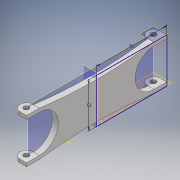
# Autodesk Inventor part: base
Saved by Autodesk Inventor 2017 (Build 210142000, 142)
## iProperties
Created: 2017-06-21
Part Number: base
Material: Generic
Document SubType Name: Modeling
Designer: erwin
Density: 1 g/cm^3
Appearance: Default
Author: erwin
Autodesk Inventor part; units mm, degrees
ref_plane "YZ Plane" through (0, 0, 0) normal (1, 0, 0) x (0, 1, 0)
ref_plane "XY Plane" through (0, 0, 0) normal (0, 0, 1) x (1, 0, 0)
ref_plane "Work Plane1" through (99, 43.8269, 0) normal (0, 0, 1) x (1, 0, 0)
sketch "Sketch1" plane through (99, 43.8269, 0) normal (0, 0, 1) x (1, 0, 0)
  circle A0 centre (13, 63.5) radius 3 projected
  arc A1 (20, 64) -> (13, 71) centre (13, 64) ccw projected
  line L0 (6, 71) -> (13, 71) projected
  arc A2 (2, 73) -> (6, 71) centre (6, 76) ccw projected
  line L1 (2, 71) -> (2, 73) projected
  line L2 (0, 71) -> (2, 71) projected
  line L3 (0, -43.8269) -> (0, 71) projected
  line L4 (-99, 0) -> (2, 0) projected
  line L5 (2, 56) -> (2, 0) projected
  line L6 (2, 56) -> (13, 56) projected
  arc A3 (13, 56) -> (20, 63) centre (13, 63) ccw projected
  line L7 (20, 64) -> (20, 63) projected
  circle A4 centre (13, 63.5) radius 3
  line L8 (6, 56) -> (21, 56)
  line L9 (21, 56) -> (21, 71)
  line L10 (21, 71) -> (6, 71)
  line L11 (6, 56) -> (20, 56)
  line L12 (20, 71) -> (6, 71)
  line L13 (6, 71) -> (6, 56)
  point P0 (-99, -43.8269)
  constraints: 12 end point, 2 horizontal, 2 parallel, 2 point on circle, 1 centre point, 1 coincident, 1 concentric, 1 perpendicular, 1 point on line
extrude "Extrusion1" add sketch "Sketch1" along normal blind 4 contours L7 A3 L6 L13 L0 A1 | A1 L10 L9 L8 A3 L7
fillet "Fillet1" radius 7 2 edges at (105, 99.8269, 2) (105, 114.8269, 2)
ref_plane "Work Plane2" through (99, 99.8269, 52) normal (0, 0, -1) x (-1, 0, 0)
sketch "Sketch2" plane through (99, 99.8269, 52) normal (0, 0, -1) x (-1, 0, 0)
  arc A0 (-6, 8) -> (-13, 15) centre (-13, 8) ccw projected
  line L0 (-21, 15) -> (-13, 15) projected
  line L1 (-21, 0) -> (-21, 15) projected
  line L2 (-13, 0) -> (-21, 0) projected
  arc A1 (-13, 0) -> (-6, 7) centre (-13, 7) ccw projected
  line L3 (-6, 8) -> (-6, 7) projected
  circle A2 centre (-13, 7.5) radius 3 projected
  point P0 (99, -99.8269)
extrude "Extrusion2" add sketch "Sketch2" along normal blind 4
sketch "Sketch3" plane through (120, 99.8269, 0) normal (1, 0, 0) x (0, 0, -1)
  line L0 (0, 15) -> (0, 8) projected
  line L1 (0, 15) -> (-52, 15)
  line L2 (-52, 15) -> (-52, -67)
  line L3 (-52, -67) -> (0, -67)
  line L4 (0, -67) -> (0, 15)
  point P0 (0, -99.8269)
  dimension "d7" = 52
  dimension "d8" = 82
  constraints: 8 end point, 2 parallel, 1 horizontal, 1 perpendicular
  measures "d7" distance of L3.end L2.end
  measures "d8" distance of L2.end L1.end
ref_plane "Work Plane3" through (120, 32.8269, 0) normal (0, 1, 0) x (-1, 0, 0)
mirror "Mirror1" about plane through (120, 32.8269, 0) normal (0, 1, 0) of "Extrusion2", "Extrusion1", "Fillet1"
sketch "Sketch4" plane through (120, -49.1731, 52) normal (1, 0, 0) x (0, 0, -1)
  line L0 (0, 7) -> (0, 0) projected
  line L1 (52, 149) -> (52, 164) projected
  line L2 (0, 0) -> (52, 0)
  line L3 (52, 0) -> (52, 164)
  line L4 (52, 164) -> (0, 164)
  line L5 (0, 164) -> (0, 0)
  point P0 (52, 49.1731)
  dimension "d9" = 164
  constraints: 8 end point, 2 parallel, 1 horizontal, 1 perpendicular
  measures "d9" distance of L1.end L2.end
extrude "Extrusion3" add sketch "Sketch4" against normal blind 2
sketch "Sketch5" plane through (118, -49.1731, 52) normal (-1, 0, 0) x (0, 0, 1)
  line L0 (34, 76) -> (-86, 76)
  line L1 (-52, 76) -> (0, 76)
  line L2 (0, 76) -> (0, 80)
  line L3 (0, 80) -> (-52, 80)
  line L4 (-52, 80) -> (-52, 76)
  line L5 (-18.5, 79.5) -> (-18.5, 80.5)
  line L6 (-33.5, 80.5) -> (-33.5, 79.5)
  line L7 (-33.5, 79.5) -> (-18.5, 80.5) construction
  line L8 (-18.5, 79.5) -> (-33.5, 80.5) construction
  arc A0 (-31.9867, 80.3991) -> (-31.9867, 79.6009) centre (-26, 80) ccw
  arc A1 (-30.9889, 80.3326) -> (-30.9889, 79.6674) centre (-26, 80) ccw
  line L9 (-31.9791, 79.5) -> (-30.9749, 79.5)
  line L10 (-21.0251, 79.5) -> (-20.0209, 79.5)
  line L11 (-20.0209, 80.5) -> (-21.0251, 80.5)
  line L12 (-30.9749, 80.5) -> (-31.9791, 80.5)
  arc A2 (-21.0251, 80.5) -> (-30.9749, 80.5) centre (-26, 80) ccw
  arc A3 (-31.9791, 79.5) -> (-20.0209, 79.5) centre (-26, 80) ccw
  arc A4 (-30.9749, 79.5) -> (-21.0251, 79.5) centre (-26, 80) ccw
  arc A5 (-21.0111, 79.6674) -> (-21.0111, 80.3326) centre (-26, 80) ccw
  arc A6 (-20.0133, 79.6009) -> (-20.0133, 80.3991) centre (-26, 80) ccw
  arc A7 (-20.0209, 80.5) -> (-31.9791, 80.5) centre (-26, 80) ccw
  point P0 (-52, 49.1731)
  dimension "d12" = 52
  dimension "d13" = 4
  dimension "d16" = 15
  dimension "d17" = 1
  constraints: 26 end point, 16 point on circle, 9 point on line, 8 centre point, 7 parallel, 4 horizontal, 3 midpoint, 3 perpendicular, 1 coincident, 2 other
  measures "d12" distance of L3.end L2.end
  measures "d13" distance of L2.end L1.end
  measures "d16" distance of L6.start L5.end
  measures "d17" distance of L5.end L5.start
extrude "Extrusion4" add sketch "Sketch5" along normal blind 12 contours A3 L0 A4 | L0 A4 L10 A3 | A3 L9 A4 L0 | L11 A2 L12 A7
sketch "Sketch6" plane through (118, -49.1731, 52) normal (-1, 0, 0) x (0, 0, 1)
  line L0 (34, 76) -> (-86, 76)
  arc A0 (-18.0156, 80.5) -> (-33.9844, 80.5) centre (-26, 80) ccw projected
  line L1 (-33.9844, 80.5) -> (-42.4844, 80.5)
  line L2 (-42.4844, 80.5) -> (-42.4844, 102.7)
  line L3 (-42.4844, 102.7) -> (-33.9844, 102.7)
  line L4 (-33.9844, 102.7) -> (-33.9844, 80.5)
  line L5 (-41.4844, 101.7) -> (-41.4844, 81.5)
  line L6 (-41.4844, 81.5) -> (-34.9844, 81.5)
  line L7 (-34.9844, 81.5) -> (-34.9844, 101.7)
  line L8 (-34.9844, 101.7) -> (-41.4844, 101.7)
  point P0 (-52, 49.1731)
  dimension "d21" = 8.5
  dimension "d22" = 22.2
  dimension "d23" = 1
  constraints: 18 end point, 4 parallel, 2 horizontal, 2 perpendicular, 5 other
  measures "d21" distance of L2.end L3.end
  measures "d22" distance of L1.end L2.end
  measures "d23" distance between parallel lines of L2 L5
extrude "Extrusion5" add sketch "Sketch6" along normal blind 10
sketch "Sketch7" plane through (118, 31.3269, 18.0156) normal (0, 0, 1) x (1, 0, 0)
  line L0 (-10, 0) -> (-10, 22.2) projected
  line L1 (0, 22.2) -> (0, 0) projected
  line L2 (-10, 11.1) -> (0, 11.1)
  line L3 (0, 11.1) -> (0, 16.1)
  line L4 (0, 16.1) -> (-10, 16.1)
  line L5 (-10, 16.1) -> (-10, 11.1)
  point P0 (-118, -31.3269)
  dimension "d26" = 5
  constraints: 8 end point, 2 parallel, 1 horizontal, 1 midpoint, 1 perpendicular, 1 point on line
  measures "d26" distance of L3.end L2.end
extrude "Extrusion6" cut sketch "Sketch7" against normal blind 1
sketch "Sketch8" plane through (118, -49.1731, 52) normal (-1, 0, 0) x (0, 0, 1)
  line L0 (-34.9844, 101.7) -> (-34.9844, 96.6) construction
  line L1 (-41.4844, 81.5) -> (-41.4844, 101.7) construction
  line L2 (-34.9844, 101.7) -> (-41.4844, 101.7) construction
  line L3 (-41.4844, 101.7) -> (-41.4844, 97.7) construction
  line L4 (-41.4844, 97.7) -> (-35.9844, 97.7) construction
  line L5 (-34.9844, 97.7) -> (-34.9844, 101.7) construction
  line L6 (-41.4844, 81.5) -> (-34.9844, 81.5) construction
  line L7 (-34.9844, 81.5) -> (-34.9844, 91.6) construction
  line L8 (-41.4844, 81.5) -> (-34.9844, 81.5) construction
  line L9 (-34.9844, 81.5) -> (-34.9844, 85.5) construction
  line L10 (-35.9844, 85.5) -> (-41.4844, 85.5) construction
  line L11 (-41.4844, 85.5) -> (-41.4844, 81.5) construction
  line L12 (-41.4844, 85.5) -> (-35.9844, 85.5)
  line L13 (-34.9844, 85.5) -> (-34.9844, 87.5)
  line L14 (-35.9844, 87.5) -> (-41.4844, 87.5)
  line L15 (-41.4844, 87.5) -> (-41.4844, 85.5)
  line L16 (-35.9844, 97.7) -> (-41.4844, 97.7)
  line L17 (-41.4844, 97.7) -> (-41.4844, 95.7)
  line L18 (-41.4844, 95.7) -> (-35.9844, 95.7)
  line L19 (-34.9844, 95.7) -> (-34.9844, 97.7)
  line L20 (-34.9844, 85.5) -> (-35.9844, 85.5)
  line L21 (-35.9844, 85.5) -> (-35.9844, 97.7)
  line L22 (-35.9844, 97.7) -> (-34.9844, 97.7)
  line L23 (-34.9844, 97.7) -> (-34.9844, 96.6)
  line L24 (-34.9844, 91.6) -> (-34.9844, 85.5)
  point P0 (-52, 49.1731)
  dimension "d29" = 4
  dimension "d30" = 4
  dimension "d31" = 2
  dimension "d32" = 2
  dimension "d36" = 1
  constraints: 44 end point, 11 parallel, 6 point on line, 5 horizontal, 5 perpendicular
  measures "d29" distance of L3.end L2.end
  measures "d30" distance of L9.end L8.end
  measures "d31" distance of L13.end L13.start
  measures "d32" distance of L17.end L16.end
  measures "d36" distance of L4.end L22.end
move faces "Move1" translate (0, -1, 0) faces at (114.6667, 47.4269, 17.6823)
extrude "Extrusion7" add sketch "Sketch8" along normal blind 3.5
sketch "Sketch9" plane through (118, -49.1731, 52) normal (-1, 0, 0) x (0, 0, 1)
  line L0 (-41.4844, 87.5) -> (-35.9844, 87.5) projected
  line L1 (-35.9844, 87.5) -> (-35.9844, 85.5) projected
  line L2 (-35.9844, 85.5) -> (-41.4844, 85.5) projected
  line L3 (-41.4844, 85.5) -> (-41.4844, 81.5) projected
  line L4 (-41.4844, 81.5) -> (-34.9844, 81.5) projected
  line L5 (-34.9844, 81.5) -> (-34.9844, 91.6) projected
  line L6 (-33.9844, 91.6) -> (-34.9844, 91.6) projected
  line L7 (-33.9844, 91.6) -> (-33.9844, 80.5) projected
  line L8 (-33.9844, 80.5) -> (-42.4844, 80.5) projected
  line L9 (-42.4844, 80.5) -> (-42.4844, 102.7) projected
  line L10 (-42.4844, 102.7) -> (-33.9844, 102.7) projected
  line L11 (-33.9844, 102.7) -> (-33.9844, 95.6) projected
  line L12 (-33.9844, 95.6) -> (-34.9844, 95.6) projected
  line L13 (-34.9844, 95.6) -> (-34.9844, 101.7) projected
  line L14 (-34.9844, 101.7) -> (-41.4844, 101.7) projected
  line L15 (-41.4844, 101.7) -> (-41.4844, 97.7) projected
  line L16 (-41.4844, 97.7) -> (-35.9844, 97.7) projected
  line L17 (-35.9844, 97.7) -> (-35.9844, 95.7) projected
  line L18 (-35.9844, 95.7) -> (-41.4844, 95.7) projected
  line L19 (-41.4844, 95.7) -> (-41.4844, 87.5) projected
  line L20 (-4, 164) -> (-4, 149) projected
  line L21 (-4, 164) -> (-48, 164) projected
  line L22 (-48, 149) -> (-48, 164) projected
  line L23 (-52, 149) -> (-48, 149) projected
  line L24 (-52, 149) -> (-52, 15) projected
  line L25 (-48, 15) -> (-52, 15) projected
  line L26 (-48, 0) -> (-48, 15) projected
  line L27 (-48, 0) -> (-4, 0) projected
  line L28 (-4, 15) -> (-4, 0) projected
  line L29 (0, 15) -> (-4, 15) projected
  line L30 (0, 15) -> (0, 149) projected
  line L31 (-4, 149) -> (0, 149) projected
  arc A0 (-20.0209, 80.5) -> (-31.9791, 80.5) centre (-26, 80) ccw projected
  line L32 (-20.0209, 80.5) -> (-21.0251, 80.5) projected
  arc A1 (-21.0251, 80.5) -> (-30.9749, 80.5) centre (-26, 80) ccw projected
  line L33 (-30.9749, 80.5) -> (-31.9791, 80.5) projected
  arc A2 (-30.9749, 79.5) -> (-21.0251, 79.5) centre (-26, 80) ccw projected
  line L34 (-21.0251, 79.5) -> (-20.0209, 79.5) projected
  arc A3 (-31.9791, 79.5) -> (-20.0209, 79.5) centre (-26, 80) ccw projected
  line L35 (-31.9791, 79.5) -> (-30.9749, 79.5) projected
  line L36 (-52, 149) -> (-48, 149) projected
  arc A4 (-48, 149) -> (-4, 149) centre (-26, 149) ccw
  arc A5 (-4, 15) -> (-48, 15) centre (-26, 15) ccw
  line L37 (0, 15) -> (-4, 15) projected
  arc A6 (0, 149) -> (0, 15) centre (495.4907, 82) ccw
  line L38 (-48, 15) -> (-52, 15) projected
  arc A7 (-52, 15) -> (-52, 149) centre (-547.4907, 82) ccw
  point P0 (-52, 49.1731)
  dimension "d39" = 22
  dimension "d40" = 22
  dimension "d41" = 500
  dimension "d42" = 500
  constraints: 8 point on circle, 4 centre point
  measures "d39" radius of A4
  measures "d40" radius of A5
  measures "d41" radius of A6
  measures "d42" radius of A7
extrude "Extrusion8" cut sketch "Sketch9" against normal blind 3.5 contours L20 A4 L22 L21 | L30 A6 | A7 L24 | L28 L27 L26 A5
sketch "Sketch10" plane through (118, -49.1731, 52) normal (-1, 0, 0) x (0, 0, 1)
  arc A0 (-30.9749, 79.5) -> (-21.0251, 79.5) centre (-26, 80) ccw projected
  line L0 (-21.0251, 79.5) -> (-20.0209, 79.5) projected
  arc A1 (-31.9791, 79.5) -> (-20.0209, 79.5) centre (-26, 80) ccw projected
  line L1 (-31.9791, 79.5) -> (-30.9749, 79.5) projected
  arc A2 (-20.0209, 80.5) -> (-31.9791, 80.5) centre (-26, 80) ccw projected
  line L2 (-20.0209, 80.5) -> (-21.0251, 80.5) projected
  arc A3 (-21.0251, 80.5) -> (-30.9749, 80.5) centre (-26, 80) ccw projected
  line L3 (-30.9749, 80.5) -> (-31.9791, 80.5) projected
  line L4 (-41.4844, 87.5) -> (-35.9844, 87.5) projected
  line L5 (-35.9844, 87.5) -> (-35.9844, 85.5) projected
  line L6 (-35.9844, 85.5) -> (-41.4844, 85.5) projected
  line L7 (-41.4844, 85.5) -> (-41.4844, 81.5) projected
  line L8 (-41.4844, 81.5) -> (-34.9844, 81.5) projected
  line L9 (-34.9844, 81.5) -> (-34.9844, 91.6) projected
  line L10 (-33.9844, 91.6) -> (-34.9844, 91.6) projected
  line L11 (-33.9844, 91.6) -> (-33.9844, 80.5) projected
  line L12 (-33.9844, 80.5) -> (-42.4844, 80.5) projected
  line L13 (-42.4844, 80.5) -> (-42.4844, 102.7) projected
  line L14 (-42.4844, 102.7) -> (-33.9844, 102.7) projected
  line L15 (-33.9844, 102.7) -> (-33.9844, 95.6) projected
  line L16 (-33.9844, 95.6) -> (-34.9844, 95.6) projected
  line L17 (-34.9844, 95.6) -> (-34.9844, 101.7) projected
  line L18 (-34.9844, 101.7) -> (-41.4844, 101.7) projected
  line L19 (-41.4844, 101.7) -> (-41.4844, 97.7) projected
  line L20 (-41.4844, 97.7) -> (-35.9844, 97.7) projected
  line L21 (-35.9844, 97.7) -> (-35.9844, 95.7) projected
  line L22 (-35.9844, 95.7) -> (-41.4844, 95.7) projected
  line L23 (-41.4844, 95.7) -> (-41.4844, 87.5) projected
  arc A4 (-48, 149) -> (-4, 149) centre (-26, 149) ccw projected
  line L24 (-52, 149) -> (-48, 149) projected
  arc A5 (-52, 15) -> (-52, 149) centre (-547.4907, 82) ccw projected
  line L25 (-48, 15) -> (-52, 15) projected
  arc A6 (-4, 15) -> (-48, 15) centre (-26, 15) ccw projected
  line L26 (0, 15) -> (-4, 15) projected
  arc A7 (0, 149) -> (0, 15) centre (495.4907, 82) ccw projected
  line L27 (-4, 149) -> (0, 149) projected
  arc A8 (-49.1869, 21.1942) -> (-49.1869, 142.8058) centre (-547.4907, 82) ccw
  arc A9 (-49.1869, 142.8058) -> (-2.8131, 142.8058) centre (-26, 149) ccw
  arc A10 (-2.8131, 142.8058) -> (-2.8131, 21.1942) centre (495.4907, 82) ccw
  arc A11 (-2.8131, 21.1942) -> (-49.1869, 21.1942) centre (-26, 15) ccw
  point P0 (-52, 49.1731)
  dimension "d45" = 2
  constraints: 8 point on circle, 4 centre point, 3 other
  measures "d45" radial gap between concentric circles of A5 A8
extrude "Extrusion9" add sketch "Sketch10" along normal blind 5 contours A4 L27 A7 L26 A6 L25 A5 L24
sketch "Sketch11" plane through (108, 46.4269, 18.0156) normal (0, -1, 0) x (1, 0, 0)
  line L0 (0, -1) -> (0, 0) projected
  line L1 (10, -1) -> (0, -1) projected
  line L2 (0, 0) -> (10, 0) projected
  line L3 (0, -1) -> (2, -1)
  line L4 (2, -1) -> (2, 0)
  line L5 (2, 0) -> (0, 0)
  line L6 (0, 0) -> (0, -1)
  point P0 (-108, -18.0156)
  dimension "d48" = 2
  constraints: 8 end point, 2 parallel, 1 horizontal, 1 perpendicular, 1 point on line
  measures "d48" distance of L5.end L4.end
extrude "Extrusion10" add sketch "Sketch11" along normal up to next
move faces "Move2" translate (3, 0, 0) faces at (110, 43.7603, 17.6823)
fillet "Fillet3" radius 2 2 edges at (113, 46.4269, 17.5156) (113, 42.4269, 17.5156)
hole "Hole1" at (118, 30.8269, 26) direction (1, 0, 0) diameter 3 depth 0.5 tip angle 118
ref_plane "Work Plane4" through (113, 32.8269, 26) normal (-1, 0, 0) x (0, -1, 0)
sketch "Sketch12" plane through (113, 32.8269, 26) normal (-1, 0, 0) x (0, -1, 0)
  line L0 (-20.7, -7.9844) -> (-20.7, -16.4844) projected
  line L1 (1.5, -7.9844) -> (-20.7, -7.9844) projected
  line L2 (-20.7, -16.4844) -> (1.5, -16.4844) projected
  line L3 (1.5, -16.4844) -> (1.5, -7.9844) projected
  arc A0 (1.5, 5.9791) -> (1.5, -5.9791) centre (2, 0) ccw projected
  arc A1 (2.5, -5.9791) -> (2.5, 5.9791) centre (2, 0) ccw projected
  line L4 (-21.7, -17.4844) -> (-21.7, -6.9844)
  line L5 (-21.7, -6.9844) -> (2.5, -6.9844)
  line L6 (2.5, -6.9844) -> (2.5, -17.4844)
  line L7 (2.5, -17.4844) -> (-21.7, -17.4844)
  arc A2 (2.4009, -5.9866) -> (1.5, -5.9791) centre (2, 0) ccw
  arc A3 (2.4009, -5.9866) -> (1.5, -5.9791) centre (2, 0) ccw
  circle A4 centre (2, 0) radius 7.0022
  line L8 (2.5, -4.9749) -> (2.5, -5.9791) projected
  circle A5 centre (2, 0) radius 6
  point P0 (32.8269, -26)
  dimension "d64" = 1
  constraints: 8 end point, 4 point on circle, 2 centre point, 2 coincident, 9 other
  measures "d64" distance between parallel lines of L0 L4
extrude "Extrusion11" add sketch "Sketch12" against normal up to next
sketch "Sketch13" plane through (118, 46.4269, 18.0156) normal (0, 0, -1) x (-1, 0, 0)
  arc A0 (3, -4) -> (3, 0) centre (3, -2) ccw projected
  line L0 (3, -4) -> (0, -4) projected
  line L1 (0, 0) -> (3, 0) projected
  line L2 (0, -4) -> (0, 0)
  point P0 (118, -46.4269)
  constraints: 2 end point, 1 vertical
extrude "Extrusion12" cut sketch "Sketch13" along normal mid plane 6
sketch "Sketch14" plane through (120, 32.8269, 547.4907) normal (1, 0, 0) x (0, 0, -1)
  point P0 (547.4907, -32.8269)
move faces "Move3" translate (3.5, 0, 0) faces at (114.5, 47.1936, 14.1823) (114.5, 37.6603, 12.349)
move faces "Move4" translate (0, 0, -0.25) faces at (110.1667, 41.0603, 10.5156) (116.8333, 47.8603, 10.5156) (110.1667, 47.1936, 10.5156) (116.8333, 37.6603, 10.5156) (110.1667, 36.9936, 10.5156) (113.5, 51.1936, 10.5156) (113.5, 33.6603, 10.5156)
move faces "Move5" translate (0, 0.25, 0) faces at (114.6667, 52.5269, 16.439) (111.3333, 52.5269, 16.0606) (111.3333, 52.5269, 10.4323) (114.6667, 52.5269, 14.1823)
move faces "Move6" translate (0, 0, 0.25) faces at (113.5183, 39.7103, 17.0156) (111.3333, 34.9936, 17.0156) (114.6667, 46.6486, 17.0156) (111.3333, 37.6603, 17.0156) (111.3333, 47.9753, 17.0156) (114.6667, 49.8603, 17.0156) (111.3333, 52.6103, 17.0156)
move faces "Move7" translate (0, -0.25, 0) faces at (114.6667, 32.3269, 16.439) (114.6667, 32.3269, 16.0606) (111.3333, 32.3269, 17.1823) (114.6667, 32.3269, 12.349) (111.3333, 32.3269, 10.349)
sketch "Sketch15" plane through (108, 31.3269, 18.0156) normal (0, 0, 1) x (1, 0, 0)
  line L0 (0, 22.2) -> (0, 0) construction
  line L1 (0, 22.2) -> (0, 18.2) construction
  point P0 (-108, -31.3269)
  dimension "d87" = 4
  constraints: 2 end point, 1 coincident, 1 point on line
  measures "d87" distance of L0.start L1.end
hole "Hole2" at (108, 49.5269, 18.0156) direction (0, 0, -1) diameter 5 depth 10
body "Solid1"
